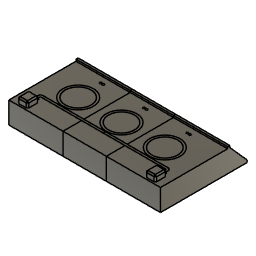
PrototypeScaleCircuit v1 (Autodesk Fusion 360 design; units mm, degrees)
Autodesk Fusion 360 part; units mm, degrees
sketch "Sketch1" plane through (0, 0, 0) normal (0, 0, 1) x (1, 0, 0)
  line L0 (-5, 0) -> (-295, 0)
  circle A0 centre (-50, 37) radius 30
  circle A1 centre (-150, 37) radius 30
  circle A2 centre (-250, 37) radius 30
  circle A3 centre (-50, 37) radius 35
  circle A4 centre (-150, 37) radius 35
  circle A5 centre (-250, 37) radius 35
  line L1 (0, -5) -> (0, -15)
  arc A6 (0, -5) -> (-5, 0) centre (-5, -5) ccw
  line L2 (-300, -5) -> (-300, -15)
  arc A7 (-295, 0) -> (-300, -5) centre (-295, -5) ccw
  line L3 (-295, -5) -> (-295, -15)
  line L4 (-5, -5) -> (-295, -5)
  line L5 (-5, -5) -> (-5, -15)
  line L6 (-300, -15) -> (-295, -15)
  line L7 (-5, -15) -> (0, -15)
  point P0 (-300, 0)
  dimension "d1" = 300
  dimension "d2" = 100
  dimension "d3" = 100
  dimension "d4" = 50
  dimension "d5" = 60
  dimension "d6" = 70
  dimension "d7" = 37
  dimension "d8" = 37
  dimension "d9" = 37
  dimension "d10" = 15
  dimension "d11" = 5
  dimension "d12" = 15
  dimension "d13" = 5
  dimension "d14" = -5
  constraint horizontal L0
  constraint concentric A0 A3
  constraint concentric A1 A4
  constraint concentric A2 A5
  constraint equal A0 A1
  constraint equal A1 A2
  constraint equal A4 A5
  constraint equal A3 A4
  constraint perpendicular L0 L1
  constraint coincident origin L0
  constraint coincident origin L1
  constraint tangent L0 A6
  constraint tangent L1 A6
  constraint perpendicular L0 L2
  constraint coincident P0 L2
  constraint coincident P0 L0
  constraint tangent L2 A7
  constraint tangent L0 A7
  constraint perpendicular L1 L7
  measures "d1" distance of origin P0
  measures "d2" distance of A0.centre A1.centre
  measures "d3" distance of A1.centre A2.centre
  measures "d4" horizontal distance of origin A0.centre
  measures "d5" diameter of A0
  measures "d6" diameter of A3
  measures "d7" distance of L0 A0.centre
  measures "d8" distance of L0 A1.centre
  measures "d9" distance of L0 A2.centre
  measures "d10" distance of origin L1.end
  measures "d11" radius of A6
  measures "d12" distance of P0 L2.end
  measures "d13" radius of A7
extrude "Extrude1" add sketch "Sketch1" along normal blind 2.2 makes body 1 at (-198.3333, -3.3333, 0) makes body 2 at (-116.9087, 33.7708, 0) makes body 3 at (-16.9087, 33.7708, 0) makes body 4 at (-216.797, 35.2612, 0)
sketch "Sketch2" plane through (0, 0, 0) normal (0, 0, -1) x (1, 0, 0)
  circle A0 centre (-50, -37) radius 30
  circle A1 centre (-50, -37) radius 35
  circle A2 centre (-150, -37) radius 30
  circle A3 centre (-150, -37) radius 35
  circle A4 centre (-250, -37) radius 30
  circle A5 centre (-250, -37) radius 35
  line L0 (-190, -77) -> (-110, -77)
  line L1 (-110, -77) -> (-110, 3)
  line L2 (-110, 3) -> (-190, 3)
  line L3 (-190, 3) -> (-190, -77)
  line L4 (-190, -77) -> (-110, 3) construction
  line L5 (-110, -77) -> (-190, 3) construction
  line L6 (-290, -77) -> (-210, -77)
  line L7 (-210, -77) -> (-210, 3)
  line L8 (-210, 3) -> (-290, 3)
  line L9 (-290, 3) -> (-290, -77)
  line L10 (-290, -77) -> (-210, 3) construction
  line L11 (-210, -77) -> (-290, 3) construction
  line L12 (-10, -77) -> (-90, -77)
  line L13 (-90, -77) -> (-90, 3)
  line L14 (-90, 3) -> (-10, 3)
  line L15 (-10, 3) -> (-10, -77)
  line L16 (-10, -77) -> (-90, 3) construction
  line L17 (-90, -77) -> (-10, 3) construction
  line L18 (-10, -37) -> (-290, -37)
  line L19 (-90, -37) -> (-10, -77)
  circle A6 centre (-50, -57) radius 2.5
  line L20 (-290, -37) -> (-210, -77)
  line L21 (-190, -37) -> (-110, -77)
  circle A7 centre (-150, -57) radius 2.5
  circle A8 centre (-250, -57) radius 2.5
  point P0 (-150, -37)
  point P1 (-250, -37)
  point P2 (-50, -37)
  dimension "d17" = 80
  dimension "d18" = 80
  dimension "d19" = 5
  constraint horizontal L0
  constraint perpendicular L0 L1
  constraint parallel L0 L2
  constraint parallel L1 L3
  constraint coincident L4 P0
  constraint coincident L5 P0
  constraint coincident P0 A2.centre
  constraint horizontal L6
  constraint perpendicular L6 L7
  constraint parallel L6 L8
  constraint parallel L7 L9
  constraint coincident L10 P1
  constraint coincident L11 P1
  constraint coincident P1 A4.centre
  constraint horizontal L12
  constraint perpendicular L12 L13
  constraint parallel L12 L14
  constraint parallel L13 L15
  constraint coincident L16 P2
  constraint coincident L17 P2
  constraint coincident P2 A0.centre
  constraint equal L1 L13
  constraint equal L3 L7
  constraint equal L0 L6
  constraint equal L0 L12
  constraint midpoint L15 L18.start
  constraint midpoint L9 L18.end
  constraint midpoint L13 L19.start
  constraint midpoint L19 A6.centre
  constraint midpoint L3 L21.start
  constraint midpoint L21 A7.centre
  constraint midpoint L20 A8.centre
  constraint equal A6 A7
  constraint equal A7 A8
  measures "d17" distance of L12.start L12.end
  measures "d18" distance of L12.start L14.end
  measures "d19" diameter of A6
extrude "Extrude2" add sketch "Sketch2" along normal blind 5 separate body contours A0 A1 L18 L19 | A0 L18 L19 A6 | A0 A1 L18 L19 | A0 A1 L19 | A0 L19 A6 | A1 L15 L18 L19 | A1 L18 L19 | A1 L12 L13 L19 | A2 A3 L18 L21 | A2 L18 L21 A7 | A2 A3 L18 L21 | A2 A3 L21 | A2 L21 A7 | A3 L1 L18 L21 | A3 L18 L21 | A3 L0 L3 L21 | A4 A5 L18 L20 | A4 L18 L20 A8 | A4 A5 L18 L20 | A4 A5 L20 | A4 L20 A8 | A5 L7 L18 L20 | A5 L18 L20 | A5 L6 L9 L20 makes body 5 at (-222.5, 57, 0) makes body 6 at (-77.5, 57, 0) makes body 7 at (-177.5, 57, 0)
sketch "Sketch3" plane through (0, 0, 0) normal (0, 0, 1) x (-1, 0, 0)
  circle A0 centre (50, -57) radius 2.5
  line L0 (10, -37) -> (10, -77)
  line L1 (10, -77) -> (90, -77)
  line L2 (90, -77) -> (90, -37)
  line L3 (90, -37) -> (10, -37)
extrude "Extrude3" add sketch "Sketch2" along normal blind 2 contours L19 A6 | L19 A6 | L21 A7 | L21 A7 | L20 A8 | L20 A8 bodies 5 6 7
sketch "Sketch4" plane through (0, -15, 0) normal (0, -1, 0) x (1, 0, 0)
  line L0 (-5, 0) -> (0, 0)
  line L1 (0, 0) -> (0, 2.2)
  line L2 (0, 2.2) -> (-5, 2.2)
  line L3 (-5, 2.2) -> (-5, 0)
  line L4 (-5, 0) -> (0, 2.2)
  circle A0 centre (-2.5, 1.1) radius 3.15
  circle A1 centre (-2.5, 1.1) radius 5.15
  line L5 (6.2794, 3.1) -> (-11.2794, 3.1)
  line L6 (-11.2794, 3.1) -> (-11.2794, -0.9)
  line L7 (-11.2794, -0.9) -> (6.2794, -0.9)
  line L8 (6.2794, -0.9) -> (6.2794, 3.1)
  line L9 (6.2794, 3.1) -> (-11.2794, -0.9) construction
  line L10 (-11.2794, 3.1) -> (6.2794, -0.9) construction
  point P0 (-2.5, 1.1)
  dimension "d24" = 6.3
  dimension "d25" = 10.3
  dimension "d26" = 4
  constraint coincident L0.start L3.end
  constraint coincident L1.end L2.start
  constraint midpoint L4 P0
  constraint concentric A0 A1
  constraint horizontal L5
  constraint perpendicular L5 L6
  constraint parallel L5 L7
  constraint parallel L6 L8
  constraint coincident L9 P0
  constraint coincident L10 P0
  constraint coincident P0 A0.centre
  measures "d24" diameter of A0
  measures "d25" diameter of A1
  measures "d26" distance of L5.start L7.end
extrude "Extrude4" add sketch "Sketch4" against normal blind 3 contours A0 L5 L7 | A0 A1 L5 L7 | A0 L5 | A0 A1 L5 | A0 A1 L7 | A0 L7 | A0 A1 L5 L7 bodies 1
extrude "Extrude5" add sketch "Sketch4" along normal blind 6 contours A0 A1 L5 L7 | A0 A1 L5 | A0 A1 L5 L7 bodies 1
extrude "Extrude6" add sketch "Sketch4" along normal blind 2 contours A0 A1 L7 bodies 1
sketch "Sketch5" plane through (0, -15, 0) normal (0, -1, 0) x (1, 0, 0)
  line L0 (-300, 0) -> (-295, 0)
  line L1 (-295, 0) -> (-295, 2.2)
  line L2 (-295, 2.2) -> (-300, 2.2)
  line L3 (-300, 2.2) -> (-300, 0)
  line L4 (-295, 2.2) -> (-300, 0)
  circle A0 centre (-297.5, 1.1) radius 3.15
  circle A1 centre (-297.5, 1.1) radius 5.15
  line L5 (-291.3228, 3.1) -> (-303.6772, 3.1)
  line L6 (-303.6772, 3.1) -> (-303.6772, -0.9)
  line L7 (-303.6772, -0.9) -> (-291.3228, -0.9)
  line L8 (-291.3228, -0.9) -> (-291.3228, 3.1)
  line L9 (-291.3228, 3.1) -> (-303.6772, -0.9) construction
  line L10 (-303.6772, 3.1) -> (-291.3228, -0.9) construction
  point P0 (-297.5, 1.1)
  dimension "d33" = 6.3
  dimension "d34" = 2
  dimension "d35" = 4
  constraint coincident L1.end L2.start
  constraint coincident L0.start L3.end
  constraint midpoint L4 P0
  constraint horizontal L5
  constraint perpendicular L5 L6
  constraint parallel L5 L7
  constraint parallel L6 L8
  constraint coincident L9 P0
  constraint coincident L10 P0
  constraint coincident P0 A0.centre
  measures "d33" diameter of A0
  measures "d35" distance of L5.start L7.end
extrude "Extrude7" add sketch "Sketch5" against normal blind 3 contours A0 L5 L7 | A0 A1 L5 L7 | A0 L5 | A0 A1 L5 | A0 A1 L7 | A0 L7 | A0 A1 L5 L7 bodies 1
extrude "Extrude8" add sketch "Sketch5" along normal blind 6 contours A0 A1 L5 L7 | A0 A1 L5 | A0 A1 L5 L7 bodies 1
extrude "Extrude9" add sketch "Sketch5" along normal blind 2 contours A0 A1 L7 bodies 1
sketch "Sketch6" plane through (0, 0, -5) normal (0, 0, -1) x (1, 0, 0)
  circle A0 centre (-50, -57) radius 2.5
  line L0 (-10, -77) -> (-10, -37)
  line L1 (-10, -37) -> (-90, -37)
  line L2 (-90, -37) -> (-90, -77)
  line L3 (-90, -77) -> (-10, -77)
  circle A1 centre (-50, -57) radius 2.5
  circle A2 centre (-150, -57) radius 2.5
  circle A3 centre (-250, -57) radius 2.5
  circle A4 centre (-50, -57) radius 4.5
  circle A5 centre (-150, -57) radius 4.5
  circle A6 centre (-250, -57) radius 4.5
  dimension "d42" = 9
  constraint concentric A1 A4
  constraint concentric A2 A5
  constraint concentric A3 A6
  constraint equal A5 A6
  constraint equal A4 A5
  measures "d42" diameter of A6
extrude "Extrude10" add sketch "Sketch6" along normal blind 4 contours A4 | A5 | A6 bodies 5 6 7
sketch "Sketch7" plane through (0, 0, 0) normal (0, 0, 1) x (-1, 0, 0)
  line L0 (10, -37) -> (10, -77)
  line L1 (10, -77) -> (90, -77)
  line L2 (90, -77) -> (90, -37)
  line L3 (90, -37) -> (10, -37)
  circle A0 centre (250, -37) radius 30
  circle A1 centre (250, -37) radius 35
  circle A2 centre (150, -37) radius 30
  circle A3 centre (150, -37) radius 30
  circle A4 centre (150, -37) radius 35
  circle A5 centre (50, -37) radius 30
  circle A6 centre (50, -37) radius 35
  line L4 (300, 12) -> (295, 12)
  line L5 (295, 12) -> (295, 5)
  line L6 (295, 5) -> (5, 5)
  line L7 (5, 5) -> (5, 12)
  line L8 (5, 12) -> (0, 12)
  line L9 (0, 12) -> (0, 5)
  arc A7 (0, 5) -> (5, 0) centre (5, 5) ccw
  line L10 (5, 0) -> (295, 0)
  arc A8 (295, 0) -> (300, 5) centre (295, 5) ccw
  line L11 (300, 5) -> (300, 12)
  line L12 (-2.65, 12) -> (7.65, 12)
  line L13 (7.2458, 17) -> (7.2458, 21)
  line L14 (7.65, 21) -> (-2.65, 21)
  line L15 (-2.2458, 21) -> (-2.2458, 17)
  line L16 (7.2458, 17) -> (-2.2458, 17)
  line L17 (292.35, 12) -> (302.65, 12)
  line L18 (302.2458, 17) -> (302.2458, 21)
  line L19 (302.65, 21) -> (292.35, 21)
  line L20 (292.7542, 21) -> (292.7542, 17)
  line L21 (302.2458, 17) -> (292.7542, 17)
  line L22 (325, -122) -> (-25, -122)
  line L23 (-25, -122) -> (-25, 48)
  line L24 (-25, 48) -> (325, 48)
  line L25 (325, 48) -> (325, -122)
  line L26 (325, -122) -> (-25, 48) construction
  line L27 (-25, -122) -> (325, 48) construction
  line L28 (11, 41) -> (-6, 41)
  line L29 (-6, 41) -> (-6, 21)
  line L30 (11, 41) -> (-6, 1) construction
  line L31 (-6, 41) -> (9.3, 5) construction
  line L32 (2.5, 21) -> (11, 21)
  line L33 (2.5, 21) -> (-6, 21)
  line L34 (-25, -112) -> (325, -112)
  line L35 (306, 41) -> (289, 41)
  line L36 (306, 21) -> (306, 41)
  line L37 (306, 41) -> (290.7, 5) construction
  line L38 (289, 41) -> (306, 1) construction
  line L39 (289, 21) -> (306, 21)
  line L40 (11, 21) -> (11, 41)
  line L41 (289, 41) -> (289, 21)
  line L42 (153, -92) -> (147, -92)
  line L43 (147, -92) -> (153, 18) construction
  circle A9 centre (153, -92) radius 2.5
  circle A10 centre (147, -92) radius 2.5
  line L44 (153, -89.5) -> (153, -92)
  line L45 (153, -92) -> (151.6339, -66.9555) construction
  line L46 (150, -37) -> (147, 18) construction
  line L47 (147, -92) -> (147, -89.5)
  circle A11 centre (53, -92) radius 2.5
  circle A12 centre (47, -92) radius 2.5
  circle A13 centre (253, -92) radius 2.5
  circle A14 centre (247, -92) radius 2.5
  circle A15 centre (50, -37) radius 29.8
  circle A16 centre (50, -37) radius 35.2
  circle A17 centre (150, -37) radius 29.8
  circle A18 centre (250, -37) radius 29.8
  circle A19 centre (250, -37) radius 35.2
  circle A20 centre (150, -37) radius 35.2
  line L48 (295, 12) -> (295, 5)
  line L49 (295, 5) -> (280, 5)
  line L50 (295, 5) -> (5, 5)
  line L51 (5.2, 5.2) -> (5.2, 12.2)
  line L52 (5.2, 12.2) -> (-0.2, 12.2)
  line L53 (-0.2, 12.2) -> (-0.2, 5)
  arc A21 (-0.2, 5) -> (5, -0.2) centre (5, 5) ccw
  line L54 (5, -0.2) -> (295, -0.2)
  arc A22 (295, -0.2) -> (300.2, 5) centre (295, 5) ccw
  line L55 (300.2, 5) -> (300.2, 12.2)
  line L56 (300.2, 12.2) -> (294.8, 12.2)
  line L57 (294.8, 12.2) -> (294.8, 5.2)
  line L58 (294.8, 5.2) -> (5.2, 5.2)
  line L59 (292.35, 12) -> (302.65, 12)
  line L60 (302.65, 12) -> (302.65, 21)
  line L61 (302.65, 21) -> (292.35, 21)
  line L62 (292.35, 21) -> (292.35, 12)
  line L63 (302.85, 21.2) -> (292.15, 21.2)
  line L64 (292.15, 21.2) -> (292.15, 11.8)
  line L65 (292.15, 11.8) -> (302.85, 11.8)
  line L66 (302.85, 11.8) -> (302.85, 21.2)
  line L67 (-2.65, 12) -> (7.65, 12)
  line L68 (7.65, 12) -> (7.65, 21)
  line L69 (7.65, 21) -> (-2.65, 21)
  line L70 (-2.65, 21) -> (-2.65, 12)
  line L71 (-2.85, 21.2) -> (-2.85, 11.8)
  line L72 (-2.85, 11.8) -> (7.85, 11.8)
  line L73 (7.85, 11.8) -> (7.85, 21.2)
  line L74 (7.85, 21.2) -> (-2.85, 21.2)
  line L75 (40, 3) -> (60, 3)
  line L76 (60, 3) -> (60, -6)
  line L77 (60, -6) -> (40, -6)
  line L78 (40, -6) -> (40, 3)
  line L79 (140, 2.7589) -> (160, 2.7589)
  line L80 (160, 2.7589) -> (160, -5.6525)
  line L81 (160, -5.6525) -> (140, -5.6525)
  line L82 (140, -5.6525) -> (140, 2.7589)
  line L83 (240, 2.7589) -> (260, 2.7589)
  line L84 (260, 2.7589) -> (260, -5.6525)
  line L85 (260, -5.6525) -> (240, -5.6525)
  line L86 (240, -5.6525) -> (240, 2.7589)
  point P0 (150, -37)
  point P1 (2.5, 21)
  point P2 (297.5, 21)
  point P3 (150, -37)
  dimension "d45" = 170
  dimension "d46" = 350
  dimension "d47" = 20
  dimension "d48" = 10
  dimension "d49" = 20
  dimension "d50" = 17
  dimension "d51" = 17
  dimension "d52" = 6
  dimension "d53" = 110
  dimension "d54" = 5
  dimension "d57" = 100
  dimension "d58" = 0
  dimension "d59" = -0.2
  dimension "d60" = 0.2
  dimension "d61" = -0.2
  dimension "d62" = -0.2
  dimension "d63" = 0.2
  dimension "d64" = 0.2
  dimension "d65" = 0.2
  dimension "d66" = 0.2
  dimension "d67" = 0.2
  dimension "d68" = 10
  dimension "d69" = 10
  dimension "d70" = 10
  dimension "d71" = 10
  dimension "d72" = 10
  dimension "d73" = 10
  constraint horizontal L22
  constraint perpendicular L22 L23
  constraint parallel L22 L24
  constraint parallel L23 L25
  constraint coincident L26 P3
  constraint coincident L27 P3
  constraint coincident P3 P0
  constraint horizontal L28
  constraint perpendicular L28 L29
  constraint coincident L30 P1
  constraint coincident L31 P1
  constraint midpoint L14 P1
  constraint coincident P1 L32.start
  constraint coincident L23 L34.start
  constraint coincident L25 L34.end
  constraint perpendicular L25 L34
  constraint horizontal L35
  constraint perpendicular L35 L41
  constraint parallel L36 L41
  constraint coincident L37 P2
  constraint coincident L38 P2
  constraint midpoint L19 P2
  constraint coincident L6 L31.end
  constraint coincident L6 L37.end
  constraint horizontal L42
  constraint perpendicular L42 L47
  constraint coincident P3 L45
  constraint coincident L43 P3
  constraint coincident L42.start A9.centre
  constraint coincident L42.end L43.start
  constraint equal A9 A10
  constraint coincident A2 L45.end
  constraint collinear L45 L46
  constraint coincident A9 L44.start
  constraint coincident A10 L47.end
  constraint coincident L4.end L5.start
  constraint coincident L5.end L6.start
  constraint coincident L6 L49.end
  constraint coincident L6.end L7.start
  constraint horizontal L59
  constraint vertical L60
  constraint horizontal L61
  constraint vertical L62
  constraint coincident L19.start L60.end
  constraint coincident L17.start L59.start
  constraint horizontal L67
  constraint vertical L68
  constraint horizontal L69
  constraint vertical L70
  constraint coincident L14.start L68.end
  constraint coincident L12.start L67.start
  constraint horizontal L75
  constraint vertical L76
  constraint horizontal L77
  constraint vertical L78
  constraint horizontal L79
  constraint vertical L80
  constraint horizontal L81
  constraint vertical L82
  constraint horizontal L83
  constraint vertical L84
  constraint horizontal L85
  constraint vertical L86
  measures "d45" distance of L22.start L24.end
  measures "d46" distance of L23.end L24.end
  measures "d47" distance of L14 L28
  measures "d48" distance of L22 L34
  measures "d49" distance of L35 P2
  measures "d50" distance of L28.start L28.end
  measures "d51" distance of L35.start L35.end
  measures "d52" distance of L42.start L42.end
  measures "d53" distance of L42.start L43.end
  measures "d54" diameter of A9
  measures "d68" distance of A5.centre L78
  measures "d69" distance of A5.centre L76
  measures "d70" distance of P3 L82
  measures "d71" distance of P3 L80
  measures "d72" distance of A0.centre L86
  measures "d73" distance of A0.centre L84
extrude "Extrude11" add sketch "Sketch7" along normal blind 2.2 separate body contours L0 L1 L2 L3 A16 | L3 A15 | L3 A15 | L23 L24 L25 L34 | A17 | A18 makes body 8 at (-43.6147, 49.703, 0) makes body 9 at (-158.1544, 27.4142, 0) makes body 10 at (-15.9959, 89.7375, 2.2) makes body 11 at (-255.451, 34.8606, 0)
sketch "Sketch8" plane through (0, 0, 0) normal (0, 0, -1) x (1, 0, 0)
  line L0 (-160, -0.2) -> (-240, -0.2)
  line L1 (-240, -0.2) -> (-240, -3.2503)
  arc A0 (-260, -3.2503) -> (-240, -3.2503) centre (-250, -37) ccw
  line L2 (-260, -3.2503) -> (-260, -0.2)
  line L3 (-260, -0.2) -> (-295, -0.2)
  arc A1 (-300.2, 5) -> (-295, -0.2) centre (-295, 5) ccw
  line L4 (-300.2, 5) -> (-300.2, 11.8)
  line L5 (-300.2, 11.8) -> (-302.85, 11.8)
  line L6 (-302.85, 11.8) -> (-302.85, 21)
  line L7 (-302.85, 21) -> (-306, 21)
  line L8 (-306, 21) -> (-306, 41)
  line L9 (-306, 41) -> (-289, 41)
  line L10 (-289, 41) -> (-289, 21)
  line L11 (-289, 21) -> (-292.15, 21)
  line L12 (-292.15, 21) -> (-292.15, 11.8)
  line L13 (-292.15, 11.8) -> (-294.8, 11.8)
  line L14 (-294.8, 11.8) -> (-294.8, 5.2)
  line L15 (-294.8, 5.2) -> (-5.2, 5.2)
  line L16 (-5.2, 5.2) -> (-5.2, 11.8)
  line L17 (-5.2, 11.8) -> (-7.85, 11.8)
  line L18 (-7.85, 11.8) -> (-7.85, 21)
  line L19 (-7.85, 21) -> (-11, 21)
  line L20 (-11, 21) -> (-11, 41)
  line L21 (-11, 41) -> (6, 41)
  line L22 (6, 41) -> (6, 21)
  line L23 (6, 21) -> (2.85, 21)
  line L24 (2.85, 21) -> (2.85, 11.8)
  line L25 (2.85, 11.8) -> (0.2, 11.8)
  line L26 (0.2, 11.8) -> (0.2, 5)
  arc A2 (-5, -0.2) -> (0.2, 5) centre (-5, 5) ccw
  line L27 (-5, -0.2) -> (-40, -0.2)
  line L28 (-40, -0.2) -> (-40, -3.2503)
  arc A3 (-60, -3.2503) -> (-40, -3.2503) centre (-50, -37) ccw
  line L29 (-60, -3.2503) -> (-60, -0.2)
  line L30 (-60, -0.2) -> (-140, -0.2)
  line L31 (-140, -0.2) -> (-140, -3.2503)
  arc A4 (-160, -3.2503) -> (-140, -3.2503) centre (-150, -37) ccw
  line L32 (-160, -3.2503) -> (-160, -0.2)
  circle A5 centre (-253, -92) radius 2.5
  circle A6 centre (-47, -92) radius 2.5
  circle A7 centre (-153, -92) radius 2.5
  circle A8 centre (-147, -92) radius 2.5
  circle A9 centre (-247, -92) radius 2.5
  circle A10 centre (-53, -92) radius 2.5
  line L33 (25, -112) -> (25, 48)
  line L34 (25, 48) -> (-325, 48)
  line L35 (-325, 48) -> (-325, -112)
  line L36 (-325, -112) -> (25, -112)
  circle A11 centre (-50, -37) radius 29.8
  circle A12 centre (-150, -37) radius 29.8
  circle A13 centre (-250, -37) radius 29.8
  circle A14 centre (-250, -57) radius 4.5
  line L37 (-210, -77) -> (-210, -37)
  line L38 (-210, -37) -> (-290, -37)
  line L39 (-290, -37) -> (-290, -77)
  line L40 (-290, -77) -> (-210, -77)
  circle A15 centre (-150, -57) radius 4.5
  line L41 (-110, -77) -> (-110, -37)
  line L42 (-110, -37) -> (-190, -37)
  line L43 (-190, -37) -> (-190, -77)
  line L44 (-190, -77) -> (-110, -77)
  circle A16 centre (-50, -57) radius 4.5
  line L45 (-10, -77) -> (-10, -37)
  line L46 (-10, -37) -> (-90, -37)
  line L47 (-90, -37) -> (-90, -77)
  line L48 (-90, -77) -> (-10, -77)
  line L49 (0.2, 11.8) -> (-5.2, 11.8)
  line L50 (-294.8, 11.8) -> (-300.2, 11.8)
  constraint coincident L25.end L26.start
  constraint coincident L16.end L17.start
  constraint coincident L13.end L14.start
  constraint coincident L4.end L5.start
extrude "Extrude12" add sketch "Sketch8" along normal blind 2 separate body contours L0 L1 A0 L2 L3 A1 L4 L14 L15 L16 L26 A2 L27 L28 A3 L29 L30 L31 A4 L32 A11 A12 A13 L38 L42 L46 L49 L50 | A12 L42 | A13 L38 | A11 L46 | L33 L34 L35 L36 picked at (-141.0504, -32.6901) picked at (-257.0661, -23.4434) picked at (-51.1836, -24.1665) makes body 12
combine "Combine1" operation add target body 12 tool bodies 8 10 9 11
sketch "Sketch9" plane through (25, 0, 0) normal (1, 0, 0) x (0, 1, 0)
  line L0 (-48, 2.2) -> (-48, -2)
  line L1 (-48, -2) -> (112, -2)
  line L2 (112, -2) -> (112, 2.2)
  line L3 (112, 2.2) -> (-48, 2.2)
  line L4 (-48, 2.2) -> (152, 2.2)
  line L5 (152, 2.2) -> (152, -47.8)
  line L6 (152, -47.8) -> (-48, -47.8)
  line L7 (-48, -47.8) -> (-48, 2.2)
  line L8 (112, 2.2) -> (152, -42.8)
  line L9 (108.263, -1.1218) -> (148.263, -46.1218)
  line L10 (152, -47.8) -> (147, -47.8)
  line L11 (147, -47.8) -> (147, -41)
  line L12 (147, -41) -> (152, -41)
  line L13 (152, -41) -> (152, -47.8)
  line L14 (-48, 2.2) -> (-43, 2.2)
  line L15 (-43, 2.2) -> (-43, -47.8)
  line L16 (-43, -47.8) -> (-48, -47.8)
  line L17 (-48, -47.8) -> (-48, 2.2)
  line L18 (-48, 2.2) -> (112, 2.2)
  line L19 (112, 2.2) -> (112, -2)
  line L20 (112, -2) -> (-48, -2)
  line L21 (-48, -2) -> (-48, 2.2)
  dimension "d78" = 50
  dimension "d79" = 40
  dimension "d80" = 5
  dimension "d81" = 5
  dimension "d82" = 5
  dimension "d83" = 5
  constraint horizontal L4
  constraint vertical L5
  constraint horizontal L6
  constraint vertical L7
  constraint coincident L0.start L3.end
  constraint coincident L2.end L3.start
  constraint coincident L5 L8.end
  constraint horizontal L10
  constraint vertical L11
  constraint horizontal L12
  constraint vertical L13
  constraint horizontal L14
  constraint vertical L15
  constraint horizontal L16
  constraint vertical L17
  constraint coincident L6 L15.end
  constraint horizontal L18
  constraint vertical L19
  constraint horizontal L20
  constraint vertical L21
  constraint coincident L1.end L2.start
  measures "d78" distance of L0.start L6.end
  measures "d79" horizontal distance of L2.end L5.end
  measures "d80" distance of L5.end L8.end
  measures "d82" distance of L11 L13
  measures "d83" distance of L15 L17
extrude "Extrude13" add sketch "Sketch9" against normal blind 350 contours L1 L6 L7 L15 L16 L17 L20 | L1 L2 L8 L9 L11 L12 L19 L20 | L5 L6 L8 L10 L11 L12 L13 bodies 12
sketch "Sketch10" plane through (25, 0, 0) normal (1, 0, 0) x (0, 1, 0)
  line L0 (-48, 2.2) -> (-48, -47.8)
  line L1 (-48, -47.8) -> (-43, -47.8)
  line L2 (-43, -47.8) -> (-43, -2)
  line L3 (-43, -2) -> (109.0436, -2)
  line L4 (109.0436, -2) -> (147, -44.701)
  line L5 (147, -44.701) -> (147, -47.8)
  line L6 (147, -47.8) -> (152, -47.8)
  line L7 (152, -47.8) -> (152, -42.8)
  line L8 (152, -42.8) -> (112, 2.2)
  line L9 (112, 2.2) -> (-48, 2.2)
  line L10 (-43, -47.8) -> (147, -47.8)
  constraint coincident L1.end L2.start
  constraint coincident L5.end L6.start
extrude "Extrude14" add sketch "Sketch10" against normal blind 4 contours L2 L3 L4 L5 L10 bodies 12
sketch "Sketch11" plane through (-325, 0, 0) normal (-1, 0, 0) x (0, -1, 0)
  line L0 (48, -47.8) -> (48, 2.2)
  line L1 (48, 2.2) -> (-112, 2.2)
  line L2 (-112, 2.2) -> (-152, -42.8)
  line L3 (-152, -42.8) -> (-152, -47.8)
  line L4 (-152, -47.8) -> (-147, -47.8)
  line L5 (-147, -47.8) -> (-147, -44.701)
  line L6 (-147, -44.701) -> (-109.0436, -2)
  line L7 (-109.0436, -2) -> (43, -2)
  line L8 (43, -2) -> (43, -47.8)
  line L9 (43, -47.8) -> (48, -47.8)
  line L10 (-147, -47.8) -> (43, -47.8)
  constraint coincident L4.end L5.start
  constraint coincident L8.end L9.start
extrude "Extrude15" add sketch "Sketch11" against normal blind 4 contours L5 L6 L7 L8 L10 bodies 12
sketch "Sketch12" plane through (0, 63.6579, 56.5848) normal (0, 0.747409, 0.664364) x (-1, 0, 0)
  line L0 (-25, -72.7644) -> (-25, -132.9724)
  line L1 (-25, -132.9724) -> (325, -132.9724)
  line L2 (325, -132.9724) -> (325, -72.7644)
  line L3 (325, -72.7644) -> (-25, -72.7644)
  line L4 (-25, -102.8684) -> (325, -102.8684)
  line L5 (70.75, -90.5684) -> (-0.75, -90.5684)
  line L6 (-0.75, -90.5684) -> (-0.75, -115.1684)
  line L7 (-0.75, -115.1684) -> (70.75, -115.1684)
  line L8 (70.75, -115.1684) -> (70.75, -90.5684)
  line L9 (70.75, -90.5684) -> (-0.75, -115.1684) construction
  line L10 (-0.75, -90.5684) -> (70.75, -115.1684) construction
  line L11 (221.25, -96.6184) -> (208.75, -96.6184)
  line L12 (208.75, -96.6184) -> (208.75, -109.1184)
  line L13 (208.75, -109.1184) -> (221.25, -109.1184)
  line L14 (221.25, -109.1184) -> (221.25, -96.6184)
  line L15 (221.25, -96.6184) -> (208.75, -109.1184) construction
  line L16 (208.75, -96.6184) -> (221.25, -109.1184) construction
  line L17 (261.25, -96.6184) -> (248.75, -96.6184)
  line L18 (248.75, -96.6184) -> (248.75, -109.1184)
  line L19 (248.75, -109.1184) -> (261.25, -109.1184)
  line L20 (261.25, -109.1184) -> (261.25, -96.6184)
  line L21 (261.25, -96.6184) -> (248.75, -109.1184) construction
  line L22 (248.75, -96.6184) -> (261.25, -109.1184) construction
  line L23 (301.25, -96.6184) -> (288.75, -96.6184)
  line L24 (288.75, -96.6184) -> (288.75, -109.1184)
  line L25 (288.75, -109.1184) -> (301.25, -109.1184)
  line L26 (301.25, -109.1184) -> (301.25, -96.6184)
  line L27 (301.25, -96.6184) -> (288.75, -109.1184) construction
  line L28 (288.75, -96.6184) -> (301.25, -109.1184) construction
  line L29 (221.25, -111.1184) -> (208.75, -111.1184)
  line L30 (208.75, -111.1184) -> (208.75, -94.6184)
  line L31 (208.75, -94.6184) -> (221.25, -94.6184)
  line L32 (221.25, -94.6184) -> (221.25, -111.1184)
  line L33 (221.25, -111.1184) -> (208.75, -94.6184) construction
  line L34 (208.75, -111.1184) -> (221.25, -94.6184) construction
  line L35 (248.75, -111.1184) -> (261.25, -111.1184)
  line L36 (261.25, -111.1184) -> (261.25, -94.6184)
  line L37 (261.25, -94.6184) -> (248.75, -94.6184)
  line L38 (248.75, -94.6184) -> (248.75, -111.1184)
  line L39 (248.75, -111.1184) -> (261.25, -94.6184) construction
  line L40 (261.25, -111.1184) -> (248.75, -94.6184) construction
  line L41 (288.75, -111.1184) -> (301.25, -111.1184)
  line L42 (301.25, -111.1184) -> (301.25, -94.6184)
  line L43 (301.25, -94.6184) -> (288.75, -94.6184)
  line L44 (288.75, -94.6184) -> (288.75, -111.1184)
  line L45 (288.75, -111.1184) -> (301.25, -94.6184) construction
  line L46 (301.25, -111.1184) -> (288.75, -94.6184) construction
  line L47 (230, -102.8684) -> (230, -95.3684)
  line L48 (230, -102.8684) -> (230, -110.3684)
  circle A0 centre (230, -95.3684) radius 2.5
  circle A1 centre (230, -110.3684) radius 2.5
  circle A2 centre (270, -110.3684) radius 2.5
  circle A3 centre (270, -95.3684) radius 2.5
  circle A4 centre (310, -110.3684) radius 2.5
  circle A5 centre (310, -95.3684) radius 2.5
  point P0 (35, -102.8684)
  point P1 (215, -102.8684)
  point P2 (255, -102.8684)
  point P3 (295, -102.8684)
  point P4 (215, -102.8684)
  point P5 (255, -102.8684)
  point P6 (295, -102.8684)
  dimension "d90" = 24.6
  dimension "d91" = 60
  dimension "d92" = 71.5
  dimension "d94" = 254.25
  dimension "d95" = 40
  dimension "d96" = 40
  dimension "d97" = 12.5
  dimension "d98" = 16.5
  dimension "d99" = 7.5
  dimension "d100" = 7.5
  dimension "d101" = 5
  dimension "d102" = 5
  dimension "d103" = 15
  dimension "d148" = 30
  dimension "d151" = 80
  dimension "d152" = 0
  constraint midpoint L0 L4.start
  constraint midpoint L2 L4.end
  constraint horizontal L5
  constraint perpendicular L5 L6
  constraint parallel L5 L7
  constraint parallel L6 L8
  constraint coincident L9 P0
  constraint coincident L10 P0
  constraint coincident L4 P0
  constraint horizontal L11
  constraint perpendicular L11 L12
  constraint parallel L11 L13
  constraint parallel L12 L14
  constraint coincident L15 P4
  constraint coincident L16 P4
  constraint coincident L4 P4
  constraint horizontal L17
  constraint perpendicular L17 L18
  constraint parallel L17 L19
  constraint parallel L18 L20
  constraint coincident L21 P5
  constraint coincident L22 P5
  constraint coincident L4 P5
  constraint horizontal L23
  constraint perpendicular L23 L24
  constraint parallel L23 L25
  constraint parallel L24 L26
  constraint coincident L27 P6
  constraint coincident L28 P6
  constraint coincident L4 P6
  constraint equal L11 L14
  constraint equal L14 L18
  constraint equal L17 L18
  constraint equal L20 L24
  constraint equal L23 L24
  constraint horizontal L29
  constraint perpendicular L29 L30
  constraint parallel L29 L31
  constraint parallel L30 L32
  constraint coincident L33 P4
  constraint coincident L34 P4
  constraint coincident P4 P1
  constraint horizontal L35
  constraint perpendicular L35 L36
  constraint parallel L35 L37
  constraint parallel L36 L38
  constraint coincident L39 P5
  constraint coincident L40 P5
  constraint coincident P5 P2
  constraint horizontal L41
  constraint perpendicular L41 L42
  constraint parallel L41 L43
  constraint parallel L42 L44
  constraint coincident L45 P6
  constraint coincident L46 P6
  constraint coincident P6 P3
  constraint equal L11 L31
  constraint equal L32 L38
  constraint equal L36 L44
  constraint equal L23 L43
  constraint equal L17 L37
  constraint coincident L4 L47.start
  constraint perpendicular L4 L47
  constraint perpendicular L4 L48
  constraint coincident L47.end A0.centre
  constraint coincident L48.end A1.centre
  measures "d90" distance of L5.end L6.end
  measures "d91" distance of L0 P0
  measures "d92" distance of L5.start L5.end
  measures "d94" distance of L2 L8
  measures "d95" distance of P4 P5
  measures "d96" distance of P5 P6
  measures "d97" distance of L11.start L11.end
  measures "d98" distance of L29.start L31.end
  measures "d99" distance of L47.start L48.end
  measures "d100" distance of L4 L47.end
  measures "d101" diameter of A0
  measures "d102" diameter of A1
  measures "d103" distance of P4 L47.start
  measures "d148" distance of L2 P6
extrude "Extrude16" cut sketch "Sketch12" against normal blind 5 contours L4 L5 L6 L8 | L4 L6 L7 L8 | L25 L41 L42 L44 | L23 L42 L43 L44 | L11 L30 L31 L32 | L13 L29 L30 L32 | L19 L35 L36 L38 | L17 L36 L37 L38 | A0 | A1 | A2 | A3 | A4 | A5 bodies 12
extrude "Extrude17" cut sketch "Sketch12" against normal blind 1 contours L4 L24 L25 L26 L42 L44 | L4 L23 L24 L26 L42 L44 | L4 L11 L12 L14 L30 L32 | L4 L12 L13 L14 L30 L32 | L4 L18 L19 L20 L36 L38 | L4 L17 L18 L20 L36 L38 bodies 12
sketch "Sketch13" plane through (0, 0, 2.2) normal (0, 0, 1) x (-1, 0, 0)
  circle A0 centre (247, -92) radius 2.5
  circle A1 centre (53, -92) radius 2.5
  circle A2 centre (153, -92) radius 2.5
  circle A3 centre (147, -92) radius 2.5
  circle A4 centre (253, -92) radius 2.5
  line L0 (240, -0.2) -> (160, -0.2)
  line L1 (160, -0.2) -> (160, -3.2503)
  arc A5 (140, -3.2503) -> (160, -3.2503) centre (150, -37) ccw
  line L2 (140, -3.2503) -> (140, -0.2)
  line L3 (140, -0.2) -> (60, -0.2)
  line L4 (60, -0.2) -> (60, -3.2503)
  arc A6 (40, -3.2503) -> (60, -3.2503) centre (50, -37) ccw
  line L5 (40, -3.2503) -> (40, -0.2)
  line L6 (40, -0.2) -> (5, -0.2)
  arc A7 (-0.2, 5) -> (5, -0.2) centre (5, 5) ccw
  line L7 (-0.2, 5) -> (-0.2, 11.8)
  line L8 (-0.2, 11.8) -> (-2.85, 11.8)
  line L9 (-2.85, 11.8) -> (-2.85, 21)
  line L10 (-2.85, 21) -> (-6, 21)
  line L11 (-6, 21) -> (-6, 41)
  line L12 (-6, 41) -> (11, 41)
  line L13 (11, 41) -> (11, 21)
  line L14 (11, 21) -> (7.85, 21)
  line L15 (7.85, 21) -> (7.85, 11.8)
  line L16 (7.85, 11.8) -> (5.2, 11.8)
  line L17 (5.2, 11.8) -> (5.2, 5.2)
  line L18 (5.2, 5.2) -> (294.8, 5.2)
  line L19 (294.8, 5.2) -> (294.8, 11.8)
  line L20 (294.8, 11.8) -> (292.15, 11.8)
  line L21 (292.15, 11.8) -> (292.15, 21)
  line L22 (292.15, 21) -> (289, 21)
  line L23 (289, 21) -> (289, 41)
  line L24 (289, 41) -> (306, 41)
  line L25 (306, 41) -> (306, 21)
  line L26 (306, 21) -> (302.85, 21)
  line L27 (302.85, 21) -> (302.85, 11.8)
  line L28 (302.85, 11.8) -> (300.2, 11.8)
  line L29 (300.2, 11.8) -> (300.2, 5)
  arc A8 (295, -0.2) -> (300.2, 5) centre (295, 5) ccw
  line L30 (295, -0.2) -> (260, -0.2)
  line L31 (260, -0.2) -> (260, -3.2503)
  arc A9 (240, -3.2503) -> (260, -3.2503) centre (250, -37) ccw
  line L32 (240, -3.2503) -> (240, -0.2)
  circle A10 centre (47, -92) radius 2.5
  line L33 (-25, 48) -> (-25, -112)
  line L34 (-25, -112) -> (325, -112)
  line L35 (325, -112) -> (325, 48)
  line L36 (325, 48) -> (-25, 48)
  line L37 (289, 21) -> (306, 21)
  line L38 (306, 21) -> (306, 41)
  line L39 (306, 41) -> (289, 41)
  line L40 (289, 41) -> (289, 21)
  line L41 (286, 18) -> (309, 18)
  line L42 (309, 18) -> (309, 44)
  line L43 (309, 44) -> (286, 44)
  line L44 (286, 44) -> (286, 18)
  line L45 (286, 21) -> (309, 21)
  line L46 (-6, 41) -> (11, 41)
  line L47 (11, 41) -> (11, 21)
  line L48 (11, 21) -> (-6, 21)
  line L49 (-6, 21) -> (-6, 41)
  line L50 (-9, 18) -> (-9, 44)
  line L51 (-9, 44) -> (14, 44)
  line L52 (14, 44) -> (14, 18)
  line L53 (14, 18) -> (-9, 18)
  line L54 (14, 21) -> (-9, 21)
  dimension "d113" = 3
  dimension "d114" = -3
  constraint horizontal L37
  constraint vertical L38
  constraint horizontal L39
  constraint vertical L40
  constraint coincident L24.end L25.start
  constraint coincident L22.end L23.start
  constraint coincident L44 L45.start
  constraint coincident L42 L45.end
  constraint perpendicular L42 L45
  constraint horizontal L46
  constraint vertical L47
  constraint horizontal L48
  constraint vertical L49
  constraint coincident L13.end L14.start
  constraint coincident L11.end L12.start
  constraint coincident L52 L54.start
  constraint coincident L50 L54.end
  constraint perpendicular L50 L54
extrude "Extrude18" add sketch "Sketch13" along normal blind 10 contours L23 L24 L25 L38 L39 L40 L42 L43 L44 L45 | L11 L12 L13 L46 L47 L49 L50 L51 L52 L54 bodies 12
sketch "Sketch14" plane through (0, 0, 12.2) normal (0, 0, 1) x (-1, 0, 0)
  line L0 (-6, 21) -> (-6, 41)
  line L1 (-6, 41) -> (11, 41)
  line L2 (11, 41) -> (11, 21)
  line L3 (11, 21) -> (14, 21)
  line L4 (14, 21) -> (14, 44)
  line L5 (14, 44) -> (-9, 44)
  line L6 (-9, 44) -> (-9, 21)
  line L7 (-9, 21) -> (-6, 21)
  line L8 (286, 44) -> (309, 44)
  line L9 (309, 44) -> (309, 21)
  line L10 (309, 21) -> (286, 21)
  line L11 (286, 21) -> (286, 44)
  line L12 (14, 44) -> (-9, 44)
  line L13 (-9, 44) -> (-9, 21)
  line L14 (-9, 21) -> (14, 21)
  line L15 (14, 21) -> (14, 44)
  constraint horizontal L8
  constraint vertical L9
  constraint horizontal L10
  constraint vertical L11
  constraint horizontal L12
  constraint vertical L13
  constraint horizontal L14
  constraint vertical L15
  constraint coincident L6.end L7.start
  constraint coincident L4.end L5.start
extrude "Extrude19" add sketch "Sketch14" along normal blind 3 bodies 12
chamfer "Chamfer1" distance 3 angle 45 5 edges at (-2.5, -44, 15.2) (9, -44, 8.7) (-14, -44, 8.7) (-14, -32.5, 15.2) (9, -32.5, 15.2) on bodies 12
chamfer "Chamfer2" distance 3 angle 45 9 edges at (-286, -32.5, 15.2) (-297.5, -44, 15.2) (-309, -32.5, 15.2) (-286, -44, 7.2) (-286, -44, 13.7) (-286, -44, 7.2) (-309, -44, 13.7) (-309, -44, 7.2) (-309, -44, 7.2) on bodies 12
sketch "Sketch15" plane through (0, 0, 2.2) normal (0, 0, 1) x (-1, 0, 0)
  line L0 (-25, 48) -> (-25, -112)
  line L1 (-25, -112) -> (325, -112)
  line L2 (325, -112) -> (325, 48)
  line L3 (325, 48) -> (-25, 48)
  circle A0 centre (47, -92) radius 2.5
  circle A1 centre (253, -92) radius 2.5
  circle A2 centre (147, -92) radius 2.5
  circle A3 centre (153, -92) radius 2.5
  circle A4 centre (53, -92) radius 2.5
  circle A5 centre (247, -92) radius 2.5
  line L4 (289, 21) -> (286, 21)
  line L5 (286, 21) -> (286, 41)
  line L6 (286, 41) -> (289, 44)
  line L7 (289, 44) -> (306, 44)
  line L8 (306, 44) -> (309, 41)
  line L9 (309, 41) -> (309, 21)
  line L10 (309, 21) -> (306, 21)
  line L11 (306, 21) -> (302.85, 21)
  line L12 (302.85, 21) -> (302.85, 11.8)
  line L13 (302.85, 11.8) -> (300.2, 11.8)
  line L14 (300.2, 11.8) -> (300.2, 5)
  arc A6 (295, -0.2) -> (300.2, 5) centre (295, 5) ccw
  line L15 (295, -0.2) -> (260, -0.2)
  line L16 (260, -0.2) -> (260, -3.2503)
  arc A7 (240, -3.2503) -> (260, -3.2503) centre (250, -37) ccw
  line L17 (240, -3.2503) -> (240, -0.2)
  line L18 (240, -0.2) -> (160, -0.2)
  line L19 (160, -0.2) -> (160, -3.2503)
  arc A8 (140, -3.2503) -> (160, -3.2503) centre (150, -37) ccw
  line L20 (140, -3.2503) -> (140, -0.2)
  line L21 (140, -0.2) -> (60, -0.2)
  line L22 (60, -0.2) -> (60, -3.2503)
  arc A9 (40, -3.2503) -> (60, -3.2503) centre (50, -37) ccw
  line L23 (40, -3.2503) -> (40, -0.2)
  line L24 (40, -0.2) -> (5, -0.2)
  arc A10 (-0.2, 5) -> (5, -0.2) centre (5, 5) ccw
  line L25 (-0.2, 5) -> (-0.2, 11.8)
  line L26 (-0.2, 11.8) -> (-2.85, 11.8)
  line L27 (-2.85, 11.8) -> (-2.85, 21)
  line L28 (-2.85, 21) -> (-6, 21)
  line L29 (-6, 21) -> (-9, 21)
  line L30 (-9, 21) -> (-9, 41)
  line L31 (-9, 41) -> (-6, 44)
  line L32 (-6, 44) -> (11, 44)
  line L33 (11, 44) -> (14, 41)
  line L34 (14, 41) -> (14, 21)
  line L35 (14, 21) -> (11, 21)
  line L36 (11, 21) -> (7.85, 21)
  line L37 (7.85, 21) -> (7.85, 11.8)
  line L38 (7.85, 11.8) -> (5.2, 11.8)
  line L39 (5.2, 11.8) -> (5.2, 5.2)
  line L40 (5.2, 5.2) -> (294.8, 5.2)
  line L41 (294.8, 5.2) -> (294.8, 11.8)
  line L42 (294.8, 11.8) -> (292.15, 11.8)
  line L43 (292.15, 11.8) -> (292.15, 21)
  line L44 (292.15, 21) -> (289, 21)
  circle A11 centre (150, -37) radius 29.8
  circle A12 centre (250, -37) radius 29.8
  circle A13 centre (50, -37) radius 29.8
  line L45 (150, -37) -> (-25, -37)
  line L46 (-25, -37) -> (325, -37)
  line L47 (-25, -37) -> (325, -37)
  line L48 (325, -37) -> (325, -112)
  line L49 (325, -112) -> (-25, -112)
  line L50 (-25, -112) -> (-25, -37)
  line L51 (325, -112) -> (-25, -112)
  line L52 (-25, -112) -> (-25, -107)
  line L53 (-25, -107) -> (325, -107)
  line L54 (325, -107) -> (325, -112)
  line L55 (325, -37) -> (-25, -37)
  line L56 (-25, -37) -> (-25, -27)
  line L57 (-25, -27) -> (325, -27)
  line L58 (325, -27) -> (325, -37)
  line L59 (325, -37) -> (-25, -37)
  line L60 (-25, -37) -> (-25, -32)
  line L61 (-25, -32) -> (325, -32)
  line L62 (325, -32) -> (325, -37)
  line L63 (325, -27) -> (292.5088, -27)
  line L64 (292.5088, -27) -> (292.5088, -32)
  line L65 (292.5088, -32) -> (325, -32)
  line L66 (325, -32) -> (325, -27)
  line L67 (325, -107) -> (-25, -107)
  line L68 (-25, -107) -> (-25, -102)
  line L69 (-25, -102) -> (325, -102)
  line L70 (325, -102) -> (325, -107)
  line L71 (325, -102) -> (320, -102)
  line L72 (320, -102) -> (320, -37)
  line L73 (320, -37) -> (325, -37)
  line L74 (325, -37) -> (325, -102)
  line L75 (-25, -102) -> (-20, -102)
  line L76 (-20, -102) -> (-20, -37)
  line L77 (-20, -37) -> (-25, -37)
  line L78 (-25, -37) -> (-25, -102)
  dimension "d121" = 5
  dimension "d122" = 10
  dimension "d123" = 5
  dimension "d126" = 5
  dimension "d127" = 5
  constraint coincident A8.centre A11.centre
  constraint coincident L0 L45.end
  constraint perpendicular L0 L45
  constraint coincident L2 L46.end
  constraint perpendicular L2 L46
  constraint horizontal L47
  constraint vertical L48
  constraint horizontal L49
  constraint vertical L50
  constraint coincident L1.end L2.start
  constraint horizontal L51
  constraint vertical L52
  constraint horizontal L53
  constraint vertical L54
  constraint horizontal L55
  constraint vertical L56
  constraint horizontal L57
  constraint vertical L58
  constraint coincident L0 L56.end
  constraint horizontal L59
  constraint vertical L60
  constraint horizontal L61
  constraint vertical L62
  constraint midpoint L56 L60.end
  constraint horizontal L63
  constraint vertical L64
  constraint horizontal L65
  constraint vertical L66
  constraint coincident L61 L64.end
  constraint horizontal L67
  constraint vertical L68
  constraint horizontal L69
  constraint vertical L70
  constraint coincident L50 L68.end
  constraint horizontal L71
  constraint vertical L72
  constraint horizontal L73
  constraint vertical L74
  constraint coincident L55 L72.end
  constraint horizontal L75
  constraint vertical L76
  constraint horizontal L77
  constraint vertical L78
  constraint coincident L45 L76.end
  measures "d121" distance of L51 L53
  measures "d122" distance of L45 L57
  measures "d123" distance of L53 L69
  measures "d126" distance of L50 L76
  measures "d127" distance of L72 L74
extrude "Extrude20" add sketch "Sketch15" along normal blind 4 contours L0 L1 L2 L48 L49 L50 L51 L52 L53 L54 L67 bodies 12
extrude "Extrude21" add sketch "Sketch15" along normal blind 10 separate body contours L0 A9 L45 L46 L47 L55 L56 L59 L60 L61 L77 | L0 L45 L46 L47 L50 L55 L59 L69 L75 L76 L77 L78 | A9 A13 L45 L46 L47 L55 L59 L61 | L2 A7 L46 L47 L55 L58 L59 L61 L62 L65 L73 | L0 L2 L48 L50 L53 L67 L68 L69 L70 L71 L75 | A13 L45 L46 L47 L55 L59 L61 | L2 L46 L47 L48 L55 L59 L69 L71 L72 L73 L74 | A9 A13 L45 L46 L47 L55 L59 L61 | A8 A9 L45 L46 L47 L55 L59 L61 | A7 A12 L46 L47 L55 L59 L61 | A8 A11 L45 L46 L47 L55 L59 L61 | A12 L46 L47 L55 L59 L61 | A8 A11 L46 L47 L55 L59 L61 | A7 A8 L46 L47 L55 L59 L61 | A11 L45 L46 L47 L55 L59 L61 | A7 A12 L46 L47 L55 L59 L61 makes body 13
sketch "Sketch16" plane through (0, 0, 12.2) normal (0, 0, 1) x (-1, 0, 0)
  line L0 (320, -37) -> (320, -102)
  line L1 (320, -102) -> (-20, -102)
  line L2 (-20, -102) -> (-20, -37)
  line L3 (-20, -37) -> (320, -37)
  line L4 (-25, -32) -> (-25, -107)
  line L5 (-25, -107) -> (325, -107)
  line L6 (325, -107) -> (325, -32)
  line L7 (325, -32) -> (-25, -32)
  line L8 (325, -69.5) -> (-25, -69.5)
  circle A0 centre (294.39, -69.5) radius 10
  circle A1 centre (0.8593, -69.5) radius 10
  dimension "d130" = 20
  dimension "d131" = 20
  constraint midpoint L6 L8.start
  constraint midpoint L4 L8.end
  constraint coincident L8 A0.centre
  constraint coincident L8 A1.centre
  measures "d130" diameter of A1
  measures "d131" diameter of A0
extrude "Extrude22" add sketch "Sketch16" along normal blind 4 contours L0 L2 L3 L4 L6 L7 L8 | L0 L2 L3 L8 A0 A1 | L0 L1 L2 L4 L5 L6 L8 | L0 L1 L2 L8 A0 A1 bodies 13
sketch "Sketch17" plane through (0, 0, -2) normal (0, 0, -1) x (1, 0, 0)
  line L0 (-321, 43) -> (-321, -109.0436)
  line L1 (-321, -109.0436) -> (21, -109.0436)
  line L2 (21, -109.0436) -> (21, 43)
  line L3 (21, 43) -> (-321, 43)
  circle A0 centre (-153, -92) radius 2.5
  circle A1 centre (-147, -92) radius 2.5
  circle A2 centre (-253, -92) radius 2.5
  circle A3 centre (-47, -92) radius 2.5
  circle A4 centre (-53, -92) radius 2.5
  circle A5 centre (-247, -92) radius 2.5
  line L4 (-10, -77) -> (-90, -77)
  line L5 (-90, -77) -> (-90, -37)
  line L6 (-90, -37) -> (-10, -37)
  line L7 (-10, -37) -> (-10, -77)
  line L8 (-110, -77) -> (-190, -77)
  line L9 (-190, -77) -> (-190, -37)
  line L10 (-190, -37) -> (-110, -37)
  line L11 (-110, -37) -> (-110, -77)
  line L12 (-292.15, 11.8) -> (-302.85, 11.8)
  line L13 (-302.85, 11.8) -> (-302.85, 21)
  line L14 (-302.85, 21) -> (-306, 21)
  line L15 (-306, 21) -> (-306, 41)
  line L16 (-306, 41) -> (-289, 41)
  line L17 (-289, 41) -> (-289, 21)
  line L18 (-289, 21) -> (-292.15, 21)
  line L19 (-292.15, 21) -> (-292.15, 11.8)
  line L20 (-210, -77) -> (-290, -77)
  line L21 (-290, -77) -> (-290, -37)
  line L22 (-290, -37) -> (-210, -37)
  line L23 (-210, -37) -> (-210, -77)
  line L24 (2.85, 11.8) -> (-7.85, 11.8)
  line L25 (-7.85, 11.8) -> (-7.85, 21)
  line L26 (-7.85, 21) -> (-11, 21)
  line L27 (-11, 21) -> (-11, 41)
  line L28 (-11, 41) -> (6, 41)
  line L29 (6, 41) -> (6, 21)
  line L30 (6, 21) -> (2.85, 21)
  line L31 (2.85, 21) -> (2.85, 11.8)
  line L32 (-167.5, 10.5) -> (-132.5, 10.5)
  line L33 (-132.5, 10.5) -> (-132.5, 25.5)
  line L34 (-132.5, 25.5) -> (-167.5, 25.5)
  line L35 (-167.5, 25.5) -> (-167.5, 10.5)
  line L36 (-167.5, 10.5) -> (-132.5, 25.5) construction
  line L37 (-132.5, 10.5) -> (-167.5, 25.5) construction
  line L38 (-169, 9.5) -> (-131, 9.5)
  line L39 (-131, 9.5) -> (-131, 11.5)
  line L40 (-131, 11.5) -> (-169, 11.5)
  line L41 (-169, 11.5) -> (-169, 9.5)
  line L42 (-169, 9.5) -> (-131, 11.5) construction
  line L43 (-131, 9.5) -> (-169, 11.5) construction
  line L44 (-169, 26.5) -> (-131, 26.5)
  line L45 (-131, 26.5) -> (-131, 24.5)
  line L46 (-131, 24.5) -> (-169, 24.5)
  line L47 (-169, 24.5) -> (-169, 26.5)
  line L48 (-169, 26.5) -> (-131, 24.5) construction
  line L49 (-131, 26.5) -> (-169, 24.5) construction
  line L50 (-171, 7.5) -> (-129, 7.5)
  line L51 (-129, 7.5) -> (-129, 13.5)
  line L52 (-129, 13.5) -> (-171, 13.5)
  line L53 (-171, 13.5) -> (-171, 7.5)
  line L54 (-171, 28.5) -> (-129, 28.5)
  line L55 (-129, 28.5) -> (-129, 22.5)
  line L56 (-129, 22.5) -> (-171, 22.5)
  line L57 (-171, 22.5) -> (-171, 28.5)
  point P0 (-150, 18)
  point P1 (-150, 10.5)
  point P2 (-150, 25.5)
  dimension "d134" = 35
  dimension "d135" = 15
  dimension "d136" = 25
  dimension "d137" = 171
  dimension "d138" = 342
  dimension "d139" = 2
  dimension "d140" = 38
  dimension "d141" = 2
  dimension "d142" = -2
  constraint horizontal L32
  constraint perpendicular L32 L33
  constraint parallel L32 L34
  constraint parallel L33 L35
  constraint coincident L36 P0
  constraint coincident L37 P0
  constraint horizontal L38
  constraint perpendicular L38 L39
  constraint parallel L38 L40
  constraint parallel L39 L41
  constraint coincident L42 P1
  constraint coincident L43 P1
  constraint midpoint L32 P1
  constraint horizontal L44
  constraint perpendicular L44 L45
  constraint parallel L44 L46
  constraint parallel L45 L47
  constraint coincident L48 P2
  constraint coincident L49 P2
  constraint midpoint L34 P2
  constraint equal L41 L47
  constraint equal L40 L46
  measures "d134" distance of L32.start L32.end
  measures "d135" distance of L32.start L34.end
  measures "d136" distance of L3 P0
  measures "d137" distance of L0 P0
  measures "d138" distance of L0.start L2.end
  measures "d139" distance of L38.start L40.end
  measures "d140" distance of L38.start L38.end
extrude "Extrude23" add sketch "Sketch17" along normal blind 8 contours L33 L35 L38 L39 L40 L41 L50 L51 L52 L53 | L33 L35 L40 L52 | L33 L35 L44 L45 L46 L47 L54 L55 L56 L57 | L33 L35 L46 L56 bodies 12
ref_plane "WorkPlane1" through (-200, 52, -20.8) normal (1, 0, 0) x (0, -1, 0)
ref_plane "WorkPlane2" through (-100, 52, -20.8) normal (1, 0, 0) x (0, -1, 0)
ref_plane "WorkPlane3" through (-150, 52, -20.8) normal (1, 0, 0) x (0, -1, 0)
split "Split1" by plane through (-150, 52, -20.8) normal (1, 0, 0) bodies 1 makes body 14 at (-101.6667, -1.6667, 0)
split "Split2" by plane through (-200, 52, -20.8) normal (1, 0, 0) bodies 12 makes body 15 at (-76.6667, -2.1667, -2)
split "Split3" by plane through (-100, 52, -20.8) normal (1, 0, 0) bodies 15 makes body 16 at (-67, -9, -2)
sketch "Sketch18" plane through (0, 0, 0) normal (1, 0, 0) x (0, 1, 0)
hidden bodies 13
equation "d1 = ( 100 * 3 ) * 1 mm"
equation "d7 = 35 mm + 2 mm"
equation "d25 = 6.3 mm + ( 2 * 2 ) * 1 mm"
equation "d98 = 12.5 mm + 4 mm"
equation "d137 = ( 342 / 2 ) * 1 mm"
equation "d145 = ( -350 / 2 ) * 1 mm - 50 mm"
equation "d146 = ( -350 / 2 ) * 1 mm + 50 mm"
equation "d147 = ( -350 / 2 ) * 1 mm"
named bodies: "MainWG", "Ring2", "Ring1", "Ring3", "BTO3", "BTO1", "BTO2", "Base", "Fluidics", "MainWG (1)", "Base (1)", "Base (1) (1)"
